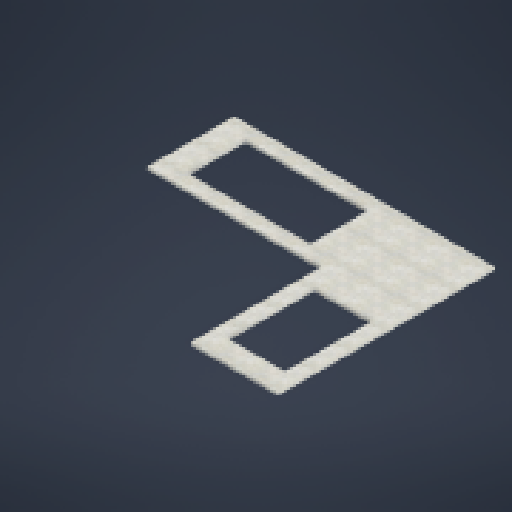
# Autodesk Inventor part: Top cucina
Saved by Autodesk Inventor 2024.2 (Build 282272000, 272)
## iProperties
Created: 2025-08-13
Part Number: Top cucina
Material: Generic
Document SubType Name: Modeling
Designer: Luca
Density: 1 g/cm^3
Appearance: Marble - Square Stacked Polished White-Brown
Author: Luca
Autodesk Inventor part; units mm, degrees
ref_plane "YZ Plane" through (0, 0, 0) normal (1, 0, 0) x (0, 1, 0)
ref_plane "XZ Plane" through (0, 0, 0) normal (0, 1, 0) x (-1, 0, 0)
ref_plane "XY Plane" through (0, 0, 0) normal (0, 0, 1) x (1, 0, 0)
sketch "Sketch1" plane through (0, 0, 0) normal (0, 1, 0) x (-1, 0, 0)
  line L0 (0, 0) -> (2150, 0)
  line L1 (2150, 0) -> (2150, 600)
  line L2 (2150, 600) -> (600, 600)
  line L3 (600, 600) -> (600, 1550)
  line L4 (600, 1550) -> (0, 1550)
  line L5 (0, 1550) -> (0, 0)
  dimension "d0" = 2150
  dimension "d1" = 600
  dimension "d2" = 1550
  constraints: 12 end point, 6 perpendicular, 1 horizontal
  measures "d0" distance of L0.start L0.end
  measures "d1" distance of L0.end L1.end
  measures "d2" distance of L4.end L0.start
extrude "Extrusion1" add sketch "Sketch1" along normal blind 20
sketch "Sketch2" plane through (0, 20, 0) normal (0, 1, 0) x (1, 0, 0)
  line L0 (-725, -500) -> (-1375, -500)
  line L1 (-1375, -500) -> (-1375, -100)
  line L2 (-1375, -100) -> (-725, -100)
  line L3 (-725, -100) -> (-725, -500)
  line L4 (-725, -500) -> (-1375, -100) construction
  line L5 (-1375, -500) -> (-725, -100) construction
  line L6 (-2150, 0) -> (-2150, -600) projected
  line L7 (0, 0) -> (-2150, 0) projected
  line L8 (-500, -1350) -> (-100, -1350)
  line L9 (-100, -1350) -> (-100, -750)
  line L10 (-100, -750) -> (-500, -750)
  line L11 (-500, -750) -> (-500, -1350)
  line L12 (-500, -1350) -> (-100, -750) construction
  line L13 (-100, -1350) -> (-500, -750) construction
  line L14 (-600, -1550) -> (0, -1550) projected
  line L15 (0, -1550) -> (0, 0) projected
  point P0 (-1050, -300)
  point P1 (-300, -1050)
  dimension "d5" = 650
  dimension "d6" = 400
  dimension "d8" = 300
  dimension "d9" = 400
  dimension "d10" = 600
  dimension "d12" = 300
  dimension "d16" = 1050
  dimension "d17" = 1050
  constraints: 24 end point, 4 midpoint, 4 parallel, 2 horizontal, 2 perpendicular
  measures "d5" distance of L1.end L2.end
  measures "d6" distance of L0.end L1.end
  measures "d8" distance from line of point (-1050, -300) L7
  measures "d9" distance of L10.end L9.end
  measures "d10" distance of L9.end L8.end
  measures "d12" distance from line of point (-300, -1050) L15
  measures "d16" distance from line of L15 point (-1050, -300)
  measures "d17" distance from line of point (-300, -1050) L7
extrude "Extrusion2" cut sketch "Sketch2" against normal through all
fillet "Fillet1" radius 20 8 edges at (-725, 10, 500) (-725, 10, 100) (-1375, 10, 100) (-1375, 10, 500) (-500, 10, 1350) (-100, 10, 1350) (-100, 10, 750) (-500, 10, 750)
body "Solid1"
